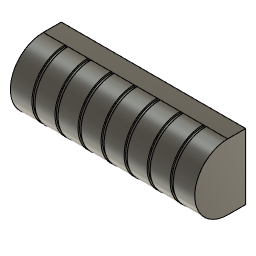
Main Body (Autodesk Fusion 360 archive; units mm, degrees)
design "Front Greeblie SM"
Autodesk Fusion 360 part; units mm, degrees
(part 1 of 2)
sketch "Sketch1" plane through (0, 0, 0) normal (1, 0, 0) x (0, 1, 0)
  circle A0 centre (0, 0) radius 2.75
  line L0 (0, 0) -> (0, 2.75) construction
  line L1 (0, 0) -> (0, -2.75) construction
  line L2 (0, 2.75) -> (1.5, 2.75)
  line L3 (1.5, 2.75) -> (1.5, -2.75)
  line L4 (1.5, -2.75) -> (0, -2.75)
  line L5 (0, -2.75) -> (0, 2.75)
  dimension "d1" = 5.5
  dimension "d42" = 1.5
  constraint coincident A0.centre L0.start
  constraint coincident A0 L0.end
  constraint vertical L0
  constraint coincident A0 L1.end
  constraint parallel L0 L1
  constraint horizontal L2
  constraint vertical L3
  constraint horizontal L4
  constraint vertical L5
  measures "d1" diameter of A0
  measures "d42" distance of L0.end L2.end
extrude "Extrude1" add sketch "Sketch1" along normal mid plane 15.4 contours A0 L5 | A0 L3 L5 | A0 L3
ref_plane "WorkPlane1" through (-7.5, 0, 0) normal (-1, 0, 0) x (0, -1, 0)
ref_plane "WorkPlane2" through (0, 0, 0) normal (1, 0, 0) x (0, 1, 0)
ref_plane "WorkPlane3" through (3.85, 0, 0) normal (1, 0, 0) x (0, 1, 0)
ref_plane "WorkPlane4" through (5.775, 0, 0) normal (1, 0, 0) x (0, 1, 0)
ref_plane "WorkPlane5" through (1.925, 0, 0) normal (1, 0, 0) x (0, 1, 0)
ref_plane "WorkPlane6" through (-3.85, 0, 0) normal (-1, 0, 0) x (0, -1, 0)
ref_plane "WorkPlane7" through (-5.775, 0, 0) normal (-1, 0, 0) x (0, -1, 0)
ref_plane "WorkPlane8" through (-1.925, 0, 0) normal (-1, 0, 0) x (0, -1, 0)
sketch "Sketch3" plane through (0, 0, 0) normal (1, 0, 0) x (0, 1, 0)
  circle A0 centre (0, 0) radius 2.75
  circle A1 centre (0, 0) radius 2.625
  dimension "d12" = 5.5
  dimension "d13" = 5.25
  constraint coincident A0.centre A1.centre
  measures "d12" diameter of A0
  measures "d13" diameter of A1
extrude "Extrude2" cut sketch "Sketch3" along normal mid plane 0.25
sketch "Sketch4" plane through (-7.5, 0, 0) normal (-1, 0, 0) x (0, 1, 0)
  circle A0 centre (0, 0) radius 2.75
  circle A1 centre (0, 0) radius 2.625
  dimension "d16" = 5.5
  dimension "d17" = 5.25
  constraint coincident A0.centre A1.centre
  constraint concentric A0 A1
  measures "d16" diameter of A0
  measures "d17" diameter of A1
sketch "Sketch5" plane through (-1.925, 0, 0) normal (-1, 0, 0) x (0, 1, 0)
  circle A0 centre (0, 0) radius 2.75
  circle A1 centre (0, 0) radius 2.625
  dimension "d18" = 5.5
  dimension "d19" = 5.25
  constraint coincident A0.centre A1.centre
  constraint concentric A0 A1
  measures "d18" diameter of A0
  measures "d19" diameter of A1
extrude "Extrude3" cut sketch "Sketch5" along normal mid plane 0.25
sketch "Sketch6" plane through (-3.85, 0, 0) normal (-1, 0, 0) x (0, 1, 0)
  circle A0 centre (0, 0) radius 2.75
  circle A1 centre (0, 0) radius 2.625
  dimension "d22" = 5.5
  dimension "d23" = 5.25
  constraint coincident A0.centre A1.centre
  measures "d22" diameter of A0
  measures "d23" diameter of A1
extrude "Extrude4" cut sketch "Sketch6" along normal mid plane 0.25
sketch "Sketch7" plane through (-5.775, 0, 0) normal (-1, 0, 0) x (0, 1, 0)
  circle A0 centre (0, 0) radius 2.75
  circle A1 centre (0, 0) radius 2.625
  dimension "d26" = 5.5
  dimension "d27" = 5.25
  constraint coincident A0.centre A1.centre
  constraint concentric A0 A1
  measures "d26" diameter of A0
  measures "d27" diameter of A1
extrude "Extrude5" cut sketch "Sketch7" along normal mid plane 0.25
sketch "Sketch8" plane through (1.925, 0, 0) normal (1, 0, 0) x (0, 1, 0)
  circle A0 centre (0, 0) radius 2.75
  circle A1 centre (0, 0) radius 2.625
  dimension "d30" = 5.5
  dimension "d31" = 5.25
  constraint coincident A0.centre A1.centre
  measures "d30" diameter of A0
  measures "d31" diameter of A1
extrude "Extrude6" cut sketch "Sketch8" along normal mid plane 0.25
sketch "Sketch9" plane through (3.85, 0, 0) normal (1, 0, 0) x (0, 1, 0)
  circle A0 centre (0, 0) radius 2.75
  circle A1 centre (0, 0) radius 2.625
  dimension "d34" = 5.5
  dimension "d35" = 5.25
  constraint coincident A0.centre A1.centre
  constraint concentric A0 A1
  measures "d34" diameter of A0
  measures "d35" diameter of A1
extrude "Extrude7" cut sketch "Sketch9" along normal mid plane 0.25
sketch "Sketch10" plane through (5.775, 0, 0) normal (1, 0, 0) x (0, 1, 0)
  circle A0 centre (0, 0) radius 2.75
  circle A1 centre (0, 0) radius 2.625
  dimension "d38" = 5.5
  dimension "d39" = 5.25
  constraint coincident A0.centre A1.centre
  constraint concentric A0 A1
  measures "d38" diameter of A0
  measures "d39" diameter of A1
extrude "Extrude8" cut sketch "Sketch10" along normal mid plane 0.25
extrude "Extrude9" add sketch "Sketch1" along normal mid plane 15.4 contours A0 L2 L3 | A0 L3 L5 | A0 L3 L4
extrude "Extrude10" cut sketch "Sketch1" along normal mid plane 20 contours A0 L3

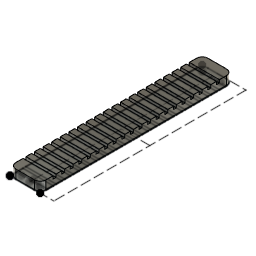
design "Panel Greeblies (v5)"
Autodesk Fusion 360 part; units mm, degrees
sketch "Sketch1" plane through (0, 0, 0) normal (0, 0, 1) x (1, 0, 0)
  line L0 (1, 0) -> (4.25, 0)
  line L1 (5.25, 1) -> (5.25, 32.5)
  line L2 (4.25, 33.5) -> (1, 33.5)
  line L3 (0, 32.5) -> (0, 1)
  arc A0 (1, 33.5) -> (0, 32.5) centre (1, 32.5) ccw
  arc A1 (5.25, 32.5) -> (4.25, 33.5) centre (4.25, 32.5) ccw
  arc A2 (4.25, 0) -> (5.25, 1) centre (4.25, 1) ccw
  arc A3 (0, 1) -> (1, 0) centre (1, 1) ccw
  line L4 (0, 1) -> (5.25, 1) construction
  line L5 (0, 32.5) -> (5.25, 32.5) construction
  line L6 (2.625, 32.5) -> (2.625, 1) construction
  line L7 (0, 32.25) -> (5.25, 32.25)
  line L8 (5.25, 32.25) -> (5.25, 31.25)
  line L9 (5.25, 31.25) -> (0, 31.25)
  line L10 (0, 31.25) -> (0, 32.25)
  line L11 (2.625, 32.5) -> (2.625, 32.25) construction
  line L12 (2.625, 1) -> (2.625, 1.42) construction
  line L13 (2.625, 31.25) -> (2.625, 30.75) construction
  line L14 (5.25, 25.25) -> (0, 25.25)
  line L15 (0, 25.25) -> (0, 26.25)
  line L16 (5.25, 26.25) -> (5.25, 25.25)
  line L17 (2.625, 25.25) -> (2.625, 24.75) construction
  line L18 (0, 26.25) -> (5.25, 26.25)
  line L19 (0, 16.25) -> (0, 17.25)
  line L20 (5.25, 17.25) -> (5.25, 16.25)
  line L21 (0, 17.25) -> (5.25, 17.25)
  line L22 (2.625, 16.25) -> (2.625, 15.75) construction
  line L23 (5.25, 16.25) -> (0, 16.25)
  line L24 (0, 7.25) -> (0, 8.25)
  line L25 (5.25, 8.25) -> (5.25, 7.25)
  line L26 (0, 8.25) -> (5.25, 8.25)
  line L27 (2.625, 7.25) -> (2.625, 6.75) construction
  line L28 (5.25, 7.25) -> (0, 7.25)
  line L29 (0, 26.75) -> (0, 27.75)
  line L30 (5.25, 27.75) -> (5.25, 26.75)
  line L31 (0, 27.75) -> (5.25, 27.75)
  line L32 (2.625, 26.75) -> (2.625, 26.25) construction
  line L33 (5.25, 26.75) -> (0, 26.75)
  line L34 (0, 22.25) -> (0, 23.25)
  line L35 (5.25, 23.25) -> (5.25, 22.25)
  line L36 (0, 23.25) -> (5.25, 23.25)
  line L37 (2.625, 22.25) -> (2.625, 21.75) construction
  line L38 (5.25, 22.25) -> (0, 22.25)
  line L39 (0, 28.25) -> (0, 29.25)
  line L40 (5.25, 29.25) -> (5.25, 28.25)
  line L41 (0, 29.25) -> (5.25, 29.25)
  line L42 (2.625, 28.25) -> (2.625, 27.75) construction
  line L43 (5.25, 28.25) -> (0, 28.25)
  line L44 (0, 13.25) -> (0, 14.25)
  line L45 (5.25, 14.25) -> (5.25, 13.25)
  line L46 (0, 14.25) -> (5.25, 14.25)
  line L47 (2.625, 13.25) -> (2.625, 12.75) construction
  line L48 (5.25, 13.25) -> (0, 13.25)
  line L49 (0, 10.25) -> (0, 11.25)
  line L50 (5.25, 11.25) -> (5.25, 10.25)
  line L51 (0, 11.25) -> (5.25, 11.25)
  line L52 (2.625, 10.25) -> (2.625, 9.75) construction
  line L53 (5.25, 10.25) -> (0, 10.25)
  line L54 (0, 11.75) -> (0, 12.75)
  line L55 (5.25, 12.75) -> (5.25, 11.75)
  line L56 (0, 12.75) -> (5.25, 12.75)
  line L57 (2.625, 11.75) -> (2.625, 11.25) construction
  line L58 (5.25, 11.75) -> (0, 11.75)
  line L59 (0, 5.75) -> (0, 6.75)
  line L60 (5.25, 6.75) -> (5.25, 5.75)
  line L61 (0, 6.75) -> (5.25, 6.75)
  line L62 (2.625, 5.75) -> (2.625, 5.25) construction
  line L63 (5.25, 5.75) -> (0, 5.75)
  line L64 (0, 17.75) -> (0, 18.75)
  line L65 (5.25, 18.75) -> (5.25, 17.75)
  line L66 (0, 18.75) -> (5.25, 18.75)
  line L67 (2.625, 17.75) -> (2.625, 17.25) construction
  line L68 (5.25, 17.75) -> (0, 17.75)
  line L69 (0, 8.75) -> (0, 9.75)
  line L70 (5.25, 9.75) -> (5.25, 8.75)
  line L71 (0, 9.75) -> (5.25, 9.75)
  line L72 (2.625, 8.75) -> (2.625, 8.25) construction
  line L73 (5.25, 8.75) -> (0, 8.75)
  line L74 (0, 29.75) -> (0, 30.75)
  line L75 (5.25, 30.75) -> (5.25, 29.75)
  line L76 (0, 30.75) -> (5.25, 30.75)
  line L77 (2.625, 29.75) -> (2.625, 29.25) construction
  line L78 (5.25, 29.75) -> (0, 29.75)
  line L79 (0, 14.75) -> (0, 15.75)
  line L80 (5.25, 15.75) -> (5.25, 14.75)
  line L81 (0, 15.75) -> (5.25, 15.75)
  line L82 (2.625, 14.75) -> (2.625, 14.25) construction
  line L83 (5.25, 14.75) -> (0, 14.75)
  line L84 (0, 19.25) -> (0, 20.25)
  line L85 (5.25, 20.25) -> (5.25, 19.25)
  line L86 (0, 20.25) -> (5.25, 20.25)
  line L87 (2.625, 19.25) -> (2.625, 18.75) construction
  line L88 (5.25, 19.25) -> (0, 19.25)
  line L89 (0, 23.75) -> (0, 24.75)
  line L90 (5.25, 24.75) -> (5.25, 23.75)
  line L91 (0, 24.75) -> (5.25, 24.75)
  line L92 (2.625, 23.75) -> (2.625, 23.25) construction
  line L93 (5.25, 23.75) -> (0, 23.75)
  line L94 (0, 20.75) -> (0, 21.75)
  line L95 (5.25, 21.75) -> (5.25, 20.75)
  line L96 (0, 21.75) -> (5.25, 21.75)
  line L97 (2.625, 20.75) -> (2.625, 20.25) construction
  line L98 (5.25, 20.75) -> (0, 20.75)
  line L99 (0, 4.25) -> (0, 5.25)
  line L100 (5.25, 5.25) -> (5.25, 4.25)
  line L101 (0, 5.25) -> (5.25, 5.25)
  line L102 (2.625, 4.25) -> (2.625, 3.75) construction
  line L103 (5.25, 4.25) -> (0, 4.25)
  line L104 (0, 2.25) -> (5.25, 2.25)
  line L105 (0, 1.25) -> (0, 2.25)
  line L106 (5.25, 1.25) -> (0, 1.25)
  line L107 (2.625, 1.25) -> (2.625, 0.75) construction
  line L108 (5.25, 2.25) -> (5.25, 1.25)
  line L109 (5.25, 2.75) -> (0, 2.75)
  line L110 (5.25, 3.75) -> (5.25, 2.75)
  line L111 (0, 3.75) -> (5.25, 3.75)
  line L112 (2.625, 2.75) -> (2.625, 2.25) construction
  line L113 (0, 2.75) -> (0, 3.75)
  line L114 (2.625, 0) -> (7.625, 0) construction
  line L115 (2.625, 33.5) -> (7.625, 33.5) construction
  line L116 (7.625, 33.5) -> (7.625, 0) construction
  line L117 (7.625, 16.75) -> (5.25, 16.75) construction
  line L118 (5.25, 16.75) -> (2.625, 16.75) construction
  point P0 (5.25, 0)
  point P1 (0, 33.5)
  dimension "d1" = 5.25
  dimension "d2" = 33.5
  dimension "d3" = 1
  dimension "d4" = 1
  dimension "d5" = 5.25
  dimension "d6" = 0.25
  dimension "d7" = 0.42
  dimension "d8" = 0.5
  dimension "d9" = 1
  dimension "d10" = 5.25
  dimension "d11" = 0.5
  dimension "d12" = 1
  dimension "d13" = 5.25
  dimension "d14" = 0.5
  dimension "d15" = 1
  dimension "d16" = 5.25
  dimension "d17" = 0.5
  dimension "d18" = 1
  dimension "d19" = 5.25
  dimension "d20" = 0.5
  dimension "d21" = 1
  dimension "d22" = 5.25
  dimension "d23" = 0.5
  dimension "d24" = 1
  dimension "d25" = 5.25
  dimension "d26" = 0.5
  dimension "d27" = 1
  dimension "d28" = 5.25
  dimension "d29" = 0.5
  dimension "d30" = 1
  dimension "d31" = 5.25
  dimension "d32" = 0.5
  dimension "d33" = 1
  dimension "d34" = 5.25
  dimension "d35" = 0.5
  dimension "d36" = 1
  dimension "d37" = 5.25
  dimension "d38" = 0.5
  dimension "d39" = 1
  dimension "d40" = 5.25
  dimension "d41" = 0.5
  dimension "d42" = 1
  dimension "d43" = 5.25
  dimension "d44" = 0.5
  dimension "d45" = 1
  dimension "d46" = 5.25
  dimension "d47" = 0.5
  dimension "d48" = 1
  dimension "d49" = 5.25
  dimension "d50" = 0.5
  dimension "d51" = 1
  dimension "d52" = 5.25
  dimension "d53" = 0.5
  dimension "d54" = 1
  dimension "d55" = 5.25
  dimension "d56" = 0.5
  dimension "d57" = 1
  dimension "d58" = 5.25
  dimension "d59" = 0.5
  dimension "d60" = 1
  dimension "d61" = 5.25
  dimension "d62" = 0.5
  dimension "d63" = 1
  dimension "d64" = 5.25
  dimension "d65" = 0.5
  dimension "d72" = 1
  dimension "d73" = 5.25
  dimension "d74" = 0.5
  dimension "d79" = 5
  dimension "d80" = 5
  constraint horizontal L0
  constraint vertical L1
  constraint horizontal L2
  constraint vertical L3
  constraint coincident P1 L3
  constraint coincident P1 L2
  constraint tangent L3 A0
  constraint tangent L2 A0
  constraint tangent L2 A1
  constraint tangent L1 A1
  constraint equal A0 A1
  constraint coincident P0 L1
  constraint coincident P0 L0
  constraint tangent L1 A2
  constraint tangent L0 A2
  constraint equal A0 A2
  constraint coincident origin L0
  constraint coincident origin L3
  constraint tangent L0 A3
  constraint tangent L3 A3
  constraint equal A0 A3
  constraint midpoint L5 L6.start
  constraint midpoint L4 L6.end
  constraint horizontal L7
  constraint vertical L8
  constraint horizontal L9
  constraint vertical L10
  constraint perpendicular L5 L11
  constraint perpendicular L4 L12
  constraint midpoint L9 L13.start
  constraint perpendicular L9 L13
  constraint horizontal L18
  constraint vertical L16
  constraint horizontal L14
  constraint vertical L15
  constraint midpoint L17.start L14
  constraint perpendicular L14 L17
  constraint midpoint L7 L11.end
  constraint horizontal L21
  constraint vertical L20
  constraint horizontal L23
  constraint vertical L19
  constraint midpoint L22.start L23
  constraint perpendicular L22 L23
  constraint horizontal L26
  constraint vertical L25
  constraint horizontal L28
  constraint vertical L24
  constraint midpoint L27.start L28
  constraint perpendicular L27 L28
  constraint horizontal L31
  constraint vertical L30
  constraint horizontal L33
  constraint vertical L29
  constraint midpoint L32.start L33
  constraint perpendicular L32 L33
  constraint horizontal L36
  constraint vertical L35
  constraint horizontal L38
  constraint vertical L34
  constraint midpoint L37.start L38
  constraint perpendicular L37 L38
  constraint horizontal L41
  constraint vertical L40
  constraint horizontal L43
  constraint vertical L39
  constraint midpoint L42.start L43
  constraint perpendicular L42 L43
  constraint horizontal L46
  constraint vertical L45
  constraint horizontal L48
  constraint vertical L44
  constraint midpoint L47.start L48
  constraint perpendicular L47 L48
  constraint horizontal L51
  constraint vertical L50
  constraint horizontal L53
  constraint vertical L49
  constraint midpoint L52.start L53
  constraint perpendicular L52 L53
  constraint horizontal L56
  constraint vertical L55
  constraint horizontal L58
  constraint vertical L54
  constraint midpoint L57.start L58
  constraint perpendicular L57 L58
  constraint horizontal L61
  constraint vertical L60
  constraint horizontal L63
  constraint vertical L59
  constraint midpoint L62.start L63
  constraint perpendicular L62 L63
  constraint horizontal L66
  constraint vertical L65
  constraint horizontal L68
  constraint vertical L64
  constraint midpoint L67.start L68
  constraint perpendicular L67 L68
  constraint horizontal L71
  constraint vertical L70
  constraint horizontal L73
  constraint vertical L69
  constraint midpoint L72.start L73
  constraint perpendicular L72 L73
  constraint horizontal L76
  constraint vertical L75
  constraint horizontal L78
  constraint vertical L74
  constraint midpoint L77.start L78
  constraint perpendicular L77 L78
  constraint horizontal L81
  constraint vertical L80
  constraint horizontal L83
  constraint vertical L79
  constraint midpoint L82.start L83
  constraint perpendicular L82 L83
  constraint horizontal L86
  constraint vertical L85
  constraint horizontal L88
  constraint vertical L84
  constraint midpoint L87.start L88
  constraint perpendicular L87 L88
  constraint horizontal L91
  constraint vertical L90
  constraint horizontal L93
  constraint vertical L89
  constraint midpoint L92.start L93
  constraint perpendicular L92 L93
  constraint horizontal L96
  constraint vertical L95
  constraint horizontal L98
  constraint vertical L94
  constraint midpoint L97.start L98
  constraint perpendicular L97 L98
  constraint horizontal L101
  constraint vertical L100
  constraint horizontal L103
  constraint vertical L99
  constraint midpoint L102.start L103
  constraint perpendicular L102 L103
  constraint midpoint L13.end L76
  constraint midpoint L41 L77.end
  constraint midpoint L31 L42.end
  constraint midpoint L18 L32.end
  constraint midpoint L17.end L91
  constraint midpoint L36 L92.end
  constraint midpoint L37.end L96
  constraint midpoint L86 L97.end
  constraint midpoint L66 L87.end
  constraint midpoint L21 L67.end
  constraint midpoint L22.end L81
  constraint midpoint L46 L82.end
  constraint midpoint L47.end L56
  constraint midpoint L51 L57.end
  constraint midpoint L52.end L71
  constraint midpoint L26 L72.end
  constraint midpoint L27.end L61
  constraint horizontal L104
  constraint vertical L108
  constraint horizontal L106
  constraint vertical L105
  constraint midpoint L107.start L106
  constraint perpendicular L106 L107
  constraint midpoint L62.end L101
  constraint horizontal L111
  constraint vertical L110
  constraint horizontal L109
  constraint vertical L113
  constraint midpoint L112.start L109
  constraint perpendicular L109 L112
  constraint midpoint L102.end L111
  constraint midpoint L104 L112.end
  constraint midpoint L0 L114.start
  constraint perpendicular L25 L114
  constraint midpoint L2 L115.start
  constraint parallel L2 L115
  constraint midpoint L116 L117.start
  constraint midpoint L20 L117.end
  constraint midpoint L6 L118.end
  measures "d1" distance of origin P0
  measures "d2" distance of origin P1
  measures "d3" radius of A0
  measures "d4" distance of L7.start L9.end
  measures "d5" distance of L8.end L9.end
  measures "d6" distance of L6.start L11.end
  measures "d7" distance of L6.end L12.end
  measures "d8" distance of L13.start L13.end
  measures "d9" distance of L14.end L15.end
  measures "d10" distance of L14.end L14.start
  measures "d11" distance of L17.start L17.end
  measures "d12" distance of L19.start L19.end
  measures "d13" distance of L19.start L20.end
  measures "d14" distance of L22.start L22.end
  measures "d15" distance of L24.start L24.end
  measures "d16" distance of L24.start L25.end
  measures "d17" distance of L27.start L27.end
  measures "d18" distance of L29.start L29.end
  measures "d19" distance of L29.start L30.end
  measures "d20" distance of L32.start L32.end
  measures "d21" distance of L34.start L34.end
  measures "d22" distance of L34.start L35.end
  measures "d23" distance of L37.start L37.end
  measures "d24" distance of L39.start L39.end
  measures "d25" distance of L39.start L40.end
  measures "d26" distance of L42.start L42.end
  measures "d27" distance of L44.start L44.end
  measures "d28" distance of L44.start L45.end
  measures "d29" distance of L47.start L47.end
  measures "d30" distance of L49.start L49.end
  measures "d31" distance of L49.start L50.end
  measures "d32" distance of L52.start L52.end
  measures "d33" distance of L54.start L54.end
  measures "d34" distance of L54.start L55.end
  measures "d35" distance of L57.start L57.end
  measures "d36" distance of L59.start L59.end
  measures "d37" distance of L59.start L60.end
  measures "d38" distance of L62.start L62.end
  measures "d39" distance of L64.start L64.end
  measures "d40" distance of L64.start L65.end
  measures "d41" distance of L67.start L67.end
  measures "d42" distance of L69.start L69.end
  measures "d43" distance of L69.start L70.end
  measures "d44" distance of L72.start L72.end
  measures "d45" distance of L74.start L74.end
  measures "d46" distance of L74.start L75.end
  measures "d47" distance of L77.start L77.end
  measures "d48" distance of L79.start L79.end
  measures "d49" distance of L79.start L80.end
  measures "d50" distance of L82.start L82.end
  measures "d51" distance of L84.start L84.end
  measures "d52" distance of L84.start L85.end
  measures "d53" distance of L87.start L87.end
  measures "d54" distance of L89.start L89.end
  measures "d55" distance of L89.start L90.end
  measures "d56" distance of L92.start L92.end
  measures "d57" distance of L94.start L94.end
  measures "d58" distance of L94.start L95.end
  measures "d59" distance of L97.start L97.end
  measures "d60" distance of L99.start L99.end
  measures "d61" distance of L99.start L100.end
  measures "d62" distance of L102.start L102.end
  measures "d63" distance of L105.start L104.start
  measures "d64" distance of L105.start L106.start
  measures "d65" distance of L107.start L107.end
  measures "d72" distance of L111.start L109.end
  measures "d73" distance of L109.start L109.end
  measures "d74" distance of L112.start L112.end
  measures "d79" distance of L114.start L114.end
  measures "d80" distance of L115.start L115.end
extrude "Extrude1" add sketch "Sketch1" along normal blind 1
extrude "Extrude2" add sketch "Sketch1" along normal blind 1.5 contours L0 L1 L3 A2 A3 L106 | L1 L3 L104 L105 L106 L108 | L1 L3 L109 L110 L111 L113 | L1 L3 L99 L100 L101 L103 | L1 L3 L59 L60 L61 L63 | L1 L3 L24 L25 L26 L28 | L1 L3 L69 L70 L71 L73 | L1 L3 L49 L50 L51 L53 | L1 L3 L54 L55 L56 L58 | L1 L3 L44 L45 L46 L48 | L1 L3 L79 L80 L81 L83 | L1 L3 L19 L20 L21 L23 | L1 L3 L64 L65 L66 L68 | L1 L3 L84 L85 L86 L88 | L1 L3 L94 L95 L96 L98 | L1 L3 L34 L35 L36 L38 | L1 L3 L89 L90 L91 L93 | L1 L3 L14 L15 L16 L18 | L1 L3 L29 L30 L31 L33 | L1 L3 L39 L40 L41 L43 | L1 L3 L74 L75 L76 L78 | L1 L3 L7 L8 L9 L10 | L1 L2 L3 A0 A1 L7

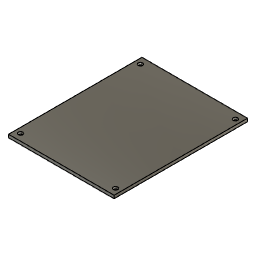
design "Back Panel (v5)"
Autodesk Fusion 360 part; units mm, degrees
sketch "Sketch1" plane through (0, 0, 0) normal (0, 0, 1) x (1, 0, 0)
  line L0 (0, 0) -> (70.25, 0)
  line L1 (70.25, 0) -> (70.25, 88.75)
  line L2 (70.25, 88.75) -> (0, 88.75)
  line L3 (0, 88.75) -> (0, 0)
  point P0 (3.5, 84.25)
  point P1 (66.75, 84.25)
  point P2 (3.5, 4.5)
  point P3 (66.75, 4.5)
  dimension "d1" = 88.75
  dimension "d2" = 70.25
  dimension "d8" = 3.5
  dimension "d9" = 4.5
  dimension "d10" = 3.5
  dimension "d11" = 4.5
  dimension "d12" = 3.5
  dimension "d13" = 4.5
  dimension "d14" = 4.5
  dimension "d15" = 3.5
  constraint horizontal L0
  constraint vertical L1
  constraint horizontal L2
  constraint vertical L3
  constraint coincident L0.start L3.end
  measures "d1" distance of L0.start L2.end
  measures "d2" distance of L0.start L0.end
  measures "d8" distance of L3 P0
  measures "d9" distance of L2 P0
  measures "d10" distance of L1 P1
  measures "d11" distance of L2 P1
  measures "d12" distance of L3 P2
  measures "d13" distance of L0 P2
  measures "d14" distance of L0 P3
  measures "d15" distance of L1 P3
extrude "Extrude1" add sketch "Sketch1" against normal blind 2
hole "Hole1" at (66.75, 84.25, 0) at (3.5, 84.25, 0) at (66.75, 4.5, 0) at (3.5, 4.5, 0) direction (0, 0, -1) diameter 1.5 end through all countersink diameter 3 countersink angle 82

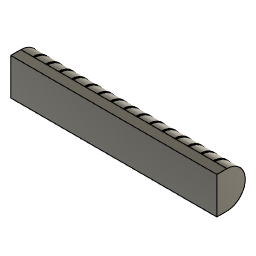
design "Front Greeblie LG"
Autodesk Fusion 360 part; units mm, degrees
sketch "Sketch1" plane through (0, 0, 0) normal (1, 0, 0) x (0, 1, 0)
  circle A0 centre (0, 0) radius 2.75
  line L0 (0, 0) -> (0, 2.75) construction
  line L1 (0, 0) -> (0, -2.75) construction
  line L2 (0, 2.75) -> (-1.5, 2.75)
  line L3 (-1.5, 2.75) -> (-1.5, -2.75)
  line L4 (-1.5, -2.75) -> (0, -2.75)
  line L5 (0, -2.75) -> (0, 2.75)
  dimension "d1" = 5.5
  dimension "d79" = 1.5
  constraint coincident A0.centre L0.start
  constraint coincident A0 L0.end
  constraint vertical L0
  constraint coincident A0 L1.end
  constraint parallel L0 L1
  constraint horizontal L2
  constraint vertical L3
  constraint horizontal L4
  constraint vertical L5
  measures "d1" diameter of A0
  measures "d79" distance of L0.end L2.end
extrude "Extrude1" add sketch "Sketch1" along normal mid plane 30.8 contours A0 L5 | A0 L3 L5 | A0 L3
ref_plane "WorkPlane1" through (0, 0, 0) normal (1, 0, 0) x (0, 1, 0)
sketch "Sketch2" plane through (0, 0, 0) normal (1, 0, 0) x (0, 1, 0)
  circle A0 centre (0, 0) radius 2.75
  circle A1 centre (0, 0) radius 2.625
  dimension "d5" = 5.5
  dimension "d6" = 5.25
  constraint coincident A0.centre A1.centre
  measures "d5" diameter of A0
  measures "d6" diameter of A1
extrude "Extrude2" cut sketch "Sketch2" along normal mid plane 0.25
ref_plane "WorkPlane2" through (7.7, 0, 0) normal (1, 0, 0) x (0, 1, 0)
sketch "Sketch3" plane through (7.7, 0, 0) normal (1, 0, 0) x (0, 1, 0)
  circle A0 centre (0, 0) radius 2.75
  circle A1 centre (0, 0) radius 2.625
  dimension "d10" = 5.5
  dimension "d11" = 5.25
  constraint coincident A0.centre A1.centre
  constraint concentric A0 A1
  measures "d10" diameter of A0
  measures "d11" diameter of A1
extrude "Extrude3" cut sketch "Sketch3" along normal mid plane 0.25
ref_plane "WorkPlane3" through (11.55, 0, 0) normal (1, 0, 0) x (0, 1, 0)
sketch "Sketch4" plane through (11.55, 0, 0) normal (1, 0, 0) x (0, 1, 0)
  circle A0 centre (0, 0) radius 2.75
  circle A1 centre (0, 0) radius 2.625
  dimension "d15" = 5.5
  dimension "d16" = 5.25
  constraint coincident A0.centre A1.centre
  constraint concentric A0 A1
  measures "d15" diameter of A0
  measures "d16" diameter of A1
extrude "Extrude4" cut sketch "Sketch4" along normal mid plane 0.25
ref_plane "WorkPlane4" through (13.475, 0, 0) normal (1, 0, 0) x (0, 1, 0)
sketch "Sketch5" plane through (13.475, 0, 0) normal (1, 0, 0) x (0, 1, 0)
  circle A0 centre (0, 0) radius 2.75
  circle A1 centre (0, 0) radius 2.625
  dimension "d20" = 5.5
  dimension "d21" = 5.25
  constraint coincident A0.centre A1.centre
  constraint concentric A0 A1
  measures "d20" diameter of A0
  measures "d21" diameter of A1
extrude "Extrude5" cut sketch "Sketch5" along normal mid plane 0.25
ref_plane "WorkPlane5" through (9.625, 0, 0) normal (1, 0, 0) x (0, 1, 0)
sketch "Sketch6" plane through (9.625, 0, 0) normal (1, 0, 0) x (0, 1, 0)
  circle A0 centre (0, 0) radius 2.75
  circle A1 centre (0, 0) radius 2.625
  dimension "d25" = 5.5
  dimension "d26" = 5.25
  constraint coincident A0.centre A1.centre
  constraint concentric A0 A1
  measures "d25" diameter of A0
  measures "d26" diameter of A1
extrude "Extrude6" cut sketch "Sketch6" along normal mid plane 0.25
ref_plane "WorkPlane6" through (5.775, 0, 0) normal (1, 0, 0) x (0, 1, 0)
sketch "Sketch7" plane through (5.775, 0, 0) normal (1, 0, 0) x (0, 1, 0)
  circle A0 centre (0, 0) radius 2.75
  circle A1 centre (0, 0) radius 2.625
  dimension "d30" = 5.5
  dimension "d31" = 5.25
  constraint coincident A0.centre A1.centre
  measures "d30" diameter of A0
  measures "d31" diameter of A1
extrude "Extrude7" cut sketch "Sketch7" along normal mid plane 0.25
ref_plane "WorkPlane7" through (3.85, 0, 0) normal (1, 0, 0) x (0, 1, 0)
sketch "Sketch8" plane through (3.85, 0, 0) normal (1, 0, 0) x (0, 1, 0)
  circle A0 centre (0, 0) radius 2.75
  circle A1 centre (0, 0) radius 2.625
  dimension "d35" = 5.5
  dimension "d36" = 5.25
  constraint coincident A0.centre A1.centre
  measures "d35" diameter of A0
  measures "d36" diameter of A1
extrude "Extrude8" cut sketch "Sketch8" along normal mid plane 0.25
ref_plane "WorkPlane8" through (1.925, 0, 0) normal (1, 0, 0) x (0, 1, 0)
sketch "Sketch9" plane through (1.925, 0, 0) normal (1, 0, 0) x (0, 1, 0)
  circle A0 centre (0, 0) radius 2.75
  circle A1 centre (0, 0) radius 2.625
  dimension "d40" = 5.5
  dimension "d41" = 5.25
  constraint coincident A0.centre A1.centre
  measures "d40" diameter of A0
  measures "d41" diameter of A1
extrude "Extrude9" cut sketch "Sketch9" along normal mid plane 0.25
ref_plane "WorkPlane9" through (-13.475, 0, 0) normal (-1, 0, 0) x (0, -1, 0)
sketch "Sketch10" plane through (-13.475, 0, 0) normal (-1, 0, 0) x (0, 1, 0)
  circle A0 centre (0, 0) radius 2.75
  circle A1 centre (0, 0) radius 2.625
  dimension "d45" = 5.5
  dimension "d46" = 5.25
  constraint coincident A0.centre A1.centre
  constraint concentric A0 A1
  measures "d45" diameter of A0
  measures "d46" diameter of A1
extrude "Extrude10" cut sketch "Sketch10" along normal mid plane 0.25
ref_plane "WorkPlane10" through (-11.55, 0, 0) normal (-1, 0, 0) x (0, -1, 0)
sketch "Sketch11" plane through (-11.55, 0, 0) normal (-1, 0, 0) x (0, 1, 0)
  circle A0 centre (0, 0) radius 2.75
  circle A1 centre (0, 0) radius 2.625
  dimension "d50" = 5.5
  dimension "d51" = 5.25
  constraint coincident A0.centre A1.centre
  measures "d50" diameter of A0
  measures "d51" diameter of A1
extrude "Extrude11" cut sketch "Sketch11" along normal mid plane 0.25
ref_plane "WorkPlane11" through (-9.625, 0, 0) normal (-1, 0, 0) x (0, -1, 0)
sketch "Sketch12" plane through (-9.625, 0, 0) normal (-1, 0, 0) x (0, 1, 0)
  circle A0 centre (0, 0) radius 2.75
  circle A1 centre (0, 0) radius 2.625
  dimension "d55" = 5.5
  dimension "d56" = 5.25
  constraint coincident A0.centre A1.centre
  constraint concentric A0 A1
  measures "d55" diameter of A0
  measures "d56" diameter of A1
extrude "Extrude12" cut sketch "Sketch12" along normal mid plane 0.25
ref_plane "WorkPlane12" through (-7.7, 0, 0) normal (-1, 0, 0) x (0, -1, 0)
sketch "Sketch13" plane through (-7.7, 0, 0) normal (-1, 0, 0) x (0, 1, 0)
  circle A0 centre (0, 0) radius 2.75
  circle A1 centre (0, 0) radius 2.625
  dimension "d60" = 5.5
  dimension "d61" = 5.25
  constraint coincident A0.centre A1.centre
  measures "d60" diameter of A0
  measures "d61" diameter of A1
extrude "Extrude13" cut sketch "Sketch13" along normal mid plane 0.25
ref_plane "WorkPlane13" through (-5.775, 0, 0) normal (-1, 0, 0) x (0, -1, 0)
sketch "Sketch14" plane through (-5.775, 0, 0) normal (-1, 0, 0) x (0, 1, 0)
  circle A0 centre (0, 0) radius 2.75
  circle A1 centre (0, 0) radius 2.625
  dimension "d65" = 5.5
  dimension "d66" = 5.25
  constraint coincident A0.centre A1.centre
  constraint concentric A0 A1
  measures "d65" diameter of A0
  measures "d66" diameter of A1
extrude "Extrude14" cut sketch "Sketch14" along normal mid plane 0.25
ref_plane "WorkPlane14" through (-3.85, 0, 0) normal (-1, 0, 0) x (0, -1, 0)
sketch "Sketch15" plane through (-3.85, 0, 0) normal (-1, 0, 0) x (0, 1, 0)
  circle A0 centre (0, 0) radius 2.75
  circle A1 centre (0, 0) radius 2.625
  dimension "d70" = 5.5
  dimension "d71" = 5.25
  constraint coincident A0.centre A1.centre
  measures "d70" diameter of A0
  measures "d71" diameter of A1
extrude "Extrude15" cut sketch "Sketch15" along normal mid plane 0.25
ref_plane "WorkPlane15" through (-1.925, 0, 0) normal (-1, 0, 0) x (0, -1, 0)
sketch "Sketch16" plane through (-1.925, 0, 0) normal (-1, 0, 0) x (0, 1, 0)
  circle A0 centre (0, 0) radius 2.75
  circle A1 centre (0, 0) radius 2.625
  dimension "d75" = 5.5
  dimension "d76" = 5.25
  constraint coincident A0.centre A1.centre
  measures "d75" diameter of A0
  measures "d76" diameter of A1
extrude "Extrude16" cut sketch "Sketch16" along normal mid plane 0.25
extrude "Extrude17" add sketch "Sketch1" along normal mid plane 30.8 contours A0 L3 L5 | A0 L2 L3 | A0 L3 L4
extrude "Extrude18" cut sketch "Sketch1" along normal mid plane 30.8 contours A0 L3

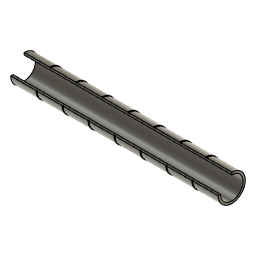
design "Front Array Greeblie"
Autodesk Fusion 360 part; units mm, degrees
sketch "Sketch1" plane through (0, 0, 0) normal (1, 0, 0) x (0, 1, 0)
  circle A0 centre (0, 0) radius 3.3
  circle A1 centre (0, 0) radius 2.75
  line L0 (0, 0) -> (-5, 0)
  line L1 (-5, 0) -> (-5, 5)
  line L2 (-5, 5) -> (0, 5)
  line L3 (0, 5) -> (0, 0)
  dimension "d1" = 6.6
  dimension "d39" = 5.5
  dimension "d42" = 5
  dimension "d43" = 5
  constraint coincident A0.centre A1.centre
  constraint concentric A0 A1
  constraint horizontal L0
  constraint vertical L1
  constraint horizontal L2
  constraint vertical L3
  measures "d1" diameter of A0
  measures "d39" diameter of A1
  measures "d42" distance of A0.centre L0.end
  measures "d43" distance of A0.centre L2.end
extrude "Extrude1" add sketch "Sketch1" along normal mid plane 50.6 contours A0 A1 L0 L3 | A0 A1 L0 L3 | A1 L0 L3 | A1 L0 L3
ref_plane "WorkPlane1" through (0, 0, 0) normal (1, 0, 0) x (0, 1, 0)
sketch "Sketch2" plane through (0, 0, 0) normal (1, 0, 0) x (0, 1, 0)
  circle A0 centre (0, 0) radius 3.3
  circle A1 centre (0, 0) radius 3.175
  dimension "d5" = 6.6
  dimension "d6" = 6.35
  constraint coincident A0.centre A1.centre
  constraint concentric A0 A1
  measures "d5" diameter of A0
  measures "d6" diameter of A1
extrude "Extrude2" cut sketch "Sketch2" along normal mid plane 0.25
ref_plane "WorkPlane2" through (12.65, 0, 0) normal (1, 0, 0) x (0, 1, 0)
sketch "Sketch3" plane through (12.65, 0, 0) normal (1, 0, 0) x (0, 1, 0)
  circle A0 centre (0, 0) radius 3.3
  circle A1 centre (0, 0) radius 3.175
  dimension "d10" = 6.6
  dimension "d11" = 6.35
  constraint coincident A0.centre A1.centre
  constraint concentric A0 A1
  measures "d10" diameter of A0
  measures "d11" diameter of A1
extrude "Extrude3" cut sketch "Sketch3" along normal mid plane 0.25
ref_plane "WorkPlane3" through (18.975, 0, 0) normal (1, 0, 0) x (0, 1, 0)
sketch "Sketch4" plane through (18.975, 0, 0) normal (1, 0, 0) x (0, 1, 0)
  circle A0 centre (0, 0) radius 3.3
  circle A1 centre (0, 0) radius 3.175
  dimension "d15" = 6.6
  dimension "d16" = 6.35
  constraint coincident A0.centre A1.centre
  constraint concentric A0 A1
  measures "d15" diameter of A0
  measures "d16" diameter of A1
extrude "Extrude4" cut sketch "Sketch4" along normal mid plane 0.25
ref_plane "WorkPlane4" through (6.325, 0, 0) normal (1, 0, 0) x (0, 1, 0)
sketch "Sketch5" plane through (6.325, 0, 0) normal (1, 0, 0) x (0, 1, 0)
  circle A0 centre (0, 0) radius 3.3
  circle A1 centre (0, 0) radius 3.175
  dimension "d20" = 6.6
  dimension "d21" = 6.35
  constraint coincident A0.centre A1.centre
  measures "d20" diameter of A0
  measures "d21" diameter of A1
extrude "Extrude5" cut sketch "Sketch5" along normal mid plane 0.25
ref_plane "WorkPlane5" through (-18.975, 0, 0) normal (-1, 0, 0) x (0, -1, 0)
sketch "Sketch6" plane through (-18.975, 0, 0) normal (-1, 0, 0) x (0, 1, 0)
  circle A0 centre (0, 0) radius 3.3
  circle A1 centre (0, 0) radius 3.175
  dimension "d25" = 6.6
  dimension "d26" = 6.35
  constraint coincident A0.centre A1.centre
  measures "d25" diameter of A0
  measures "d26" diameter of A1
extrude "Extrude6" cut sketch "Sketch6" along normal mid plane 0.25
ref_plane "WorkPlane6" through (-12.65, 0, 0) normal (-1, 0, 0) x (0, -1, 0)
sketch "Sketch7" plane through (-12.65, 0, 0) normal (-1, 0, 0) x (0, 1, 0)
  circle A0 centre (0, 0) radius 3.3
  circle A1 centre (0, 0) radius 3.175
  dimension "d30" = 6.6
  dimension "d31" = 6.35
  constraint coincident A0.centre A1.centre
  measures "d30" diameter of A0
  measures "d31" diameter of A1
extrude "Extrude7" cut sketch "Sketch7" along normal mid plane 0.25
ref_plane "WorkPlane7" through (-6.325, 0, 0) normal (-1, 0, 0) x (0, -1, 0)
sketch "Sketch8" plane through (-6.325, 0, 0) normal (-1, 0, 0) x (0, 1, 0)
  circle A0 centre (0, 0) radius 3.3
  circle A1 centre (0, 0) radius 3.175
  dimension "d35" = 6.6
  dimension "d36" = 6.35
  constraint coincident A0.centre A1.centre
  measures "d35" diameter of A0
  measures "d36" diameter of A1
extrude "Extrude8" cut sketch "Sketch8" along normal mid plane 0.25
extrude "Extrude9" cut sketch "Sketch1" along normal mid plane 60 contours A1 L0 L3 | A1 L0 L3
extrude "Extrude10" cut sketch "Sketch1" along normal mid plane 60 contours A0 A1 L0 L3 picked at (-3.1055, 0.1565)

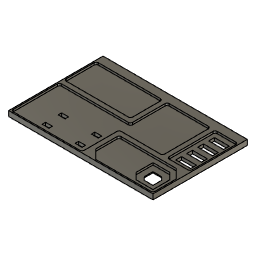
design "Lower Interface (v5)"
Autodesk Fusion 360 part; units mm, degrees